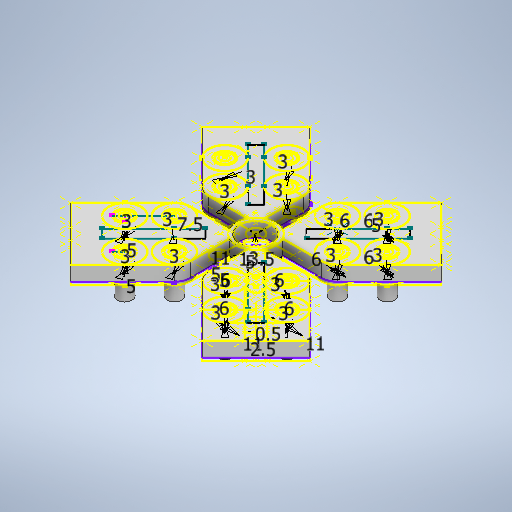
# Autodesk Inventor part: Gripper_Gen3_Base
Saved by Autodesk Inventor 2025.1 (Build 291241000, 241)
## iProperties
Created: 2024-10-29
Part Number: Gripper_Gen3_Base
Material: Generic
Document SubType Name: Modeling
Designer: m_kni
Density: 1 g/cm^3
Appearance: Default
Author: m_kni
Autodesk Inventor part; units mm, degrees
(part 1 of 3)
ref_plane "YZ Plane" through (0, 0, 0) normal (1, 0, 0) x (0, 1, 0)
ref_plane "XZ Plane" through (0, 0, 0) normal (0, 1, 0) x (-1, 0, 0)
ref_plane "XY Plane" through (0, 0, 0) normal (0, 0, 1) x (1, 0, 0)
sketch "Sketch1" plane through (0, 0, 0) normal (0, 1, 0) x (-1, 0, 0)
  arc A0 (-14.3226, 10.9666) -> (-12.7316, 10.3076) centre (-12.7316, 12.5576) ccw
  arc A1 (-14.3226, 10.9666) -> (-12.7316, 10.3076) centre (-12.7316, 12.5576) ccw
  line L0 (-12.7316, 10.3076) -> (-12.7316, 12.5576)
  line L1 (-12.7316, 10.3076) -> (-12.7316, 12.5576)
  line L2 (-12.7316, 12.5576) -> (-10.4816, 12.5576)
  line L3 (-12.7316, 12.5576) -> (-10.4816, 12.5576)
  arc A2 (-14.3226, 17.3306) -> (-17.5046, 14.1486) centre (-15.9136, 15.7396) ccw
  line L4 (-17.5046, 14.1486) -> (-14.3226, 10.9666)
  line L5 (-11.1407, 14.1486) -> (-14.3226, 17.3306)
  arc A3 (-10.4816, 12.5576) -> (-11.1407, 14.1486) centre (-12.7316, 12.5576) ccw
  arc A4 (-14.3226, 17.3306) -> (-17.5046, 14.1486) centre (-15.9136, 15.7396) ccw
  line L6 (-22.9847, 25.9926) -> (-14.3226, 17.3306)
  line L7 (-17.5046, 14.1486) -> (-26.1667, 22.8107)
  arc A5 (-10.4816, 12.5576) -> (-11.1407, 14.1486) centre (-12.7316, 12.5576) ccw
  line L8 (-26.1667, 22.8107) -> (-14.3226, 10.9666)
  line L9 (-26.1667, 22.8107) -> (-14.3226, 10.9666)
  line L10 (-25.9899, 22.9874) -> (-26.1667, 22.8107)
  line L11 (-22.9847, 25.9926) -> (-26.1667, 22.8107)
  line L12 (-26.1667, 22.8107) -> (-22.9847, 25.9926)
  line L13 (-11.1407, 14.1486) -> (-22.9847, 25.9926)
  arc A6 (-10.5886, 13.2429) -> (-11.1407, 14.1486) centre (-12.7316, 12.5576) ccw
  arc A7 (-14.3226, 10.9666) -> (-13.417, 10.4145) centre (-12.7316, 12.5576) ccw
  line L14 (-23.1615, 25.8159) -> (-10.5886, 13.2429)
  line L15 (-22.9847, 25.9926) -> (-11.1407, 14.1486)
  line L16 (-23.1615, 25.8159) -> (-22.9847, 25.9926)
  line L17 (-25.9899, 22.9874) -> (-13.417, 10.4145)
  line L18 (-14.3226, 10.9666) -> (-26.1667, 22.8107)
  line L19 (-26.1667, 22.8107) -> (-25.9899, 22.9874)
  arc A8 (-14.3226, 10.9666) -> (-13.417, 10.4145) centre (-12.7316, 12.5576) ccw
  arc A9 (-10.5886, 13.2429) -> (-11.1407, 14.1486) centre (-12.7316, 12.5576) ccw
  line L20 (-23.1615, 25.8159) -> (-10.5886, 13.2429)
  line L21 (-11.1407, 14.1486) -> (-22.9847, 25.9926)
  line L22 (-22.9847, 25.9926) -> (-23.1615, 25.8159)
  circle A10 centre (-19.2671, 8.4864) radius 2.5
  circle A11 centre (-19.2671, 8.4864) radius 2.5
  circle A12 centre (-17.1458, 27.5783) radius 2.5
  circle A13 centre (-17.1458, 27.5783) radius 2.5
  circle A14 centre (-8.6605, 19.0931) radius 5.5
  circle A15 centre (-27.7524, 16.9717) radius 2.5
  circle A16 centre (-27.7524, 16.9717) radius 2.5
  line L23 (-20.5045, 20.3305) -> (-23.3382, 23.1642)
  arc A17 (-14.3226, 17.3306) -> (-18.0567, 15.0542) centre (-15.9136, 15.7396) ccw
  line L24 (-12.7316, 10.3076) -> (-12.7316, 12.5576)
  line L25 (-12.7316, 12.5576) -> (-10.4816, 12.5576)
  arc A18 (-14.3226, 10.9666) -> (-12.7316, 10.3076) centre (-12.7316, 12.5576) ccw
  arc A19 (-10.4816, 12.5576) -> (-11.1407, 14.1486) centre (-12.7316, 12.5576) ccw
  line L26 (-27.7524, 16.9717) -> (-31.6415, 13.0826)
  line L27 (-31.6415, 13.0826) -> (-23.1562, 4.5974)
  line L28 (-17.1458, 27.5783) -> (-13.2567, 31.4674)
  line L29 (-13.2567, 31.4674) -> (-4.7714, 22.9821)
  circle A20 centre (-0.0316, 12.5576) radius 2.5
  line L30 (-20.5045, 20.3305) -> (-23.3382, 23.1642)
  line L31 (-6.1605, 19.0931) -> (-3.1605, 19.0931)
  line L32 (-3.1605, 19.0931) -> (-3.1605, 12.6302)
  circle A21 centre (-0.0316, -0.1424) radius 6.75
  circle A22 centre (-0.0316, -0.1424) radius 2.5
  line L33 (-3.1605, 12.6302) -> (-3.1605, 5.8386)
  line L34 (-0.0316, -0.1424) -> (-12.7316, -0.1424)
  line L35 (-0.0316, -0.1424) -> (-0.0316, 12.5576)
  line L36 (-0.0316, -0.1424) -> (12.6684, -0.1424)
  line L37 (-19.2671, 2.9864) -> (-6.0127, 2.9864)
  circle A23 centre (-0.0316, -0.1424) radius 2.5
  line L38 (-0.0316, -0.1424) -> (-0.0316, -12.8424)
  line L39 (-20.5045, 24.2196) -> (-13.9798, 17.6948)
  line L40 (-24.3936, 20.3305) -> (-29.7263, 25.6631)
  line L41 (-24.3936, 20.3305) -> (-16.8521, 20.3305) construction
  line L42 (-20.5045, 24.2196) -> (-25.8372, 29.5522)
  line L43 (-29.7263, 25.6631) -> (-33.6153, 29.5522)
  line L44 (-33.6153, 29.5522) -> (-29.7263, 33.4413)
  line L45 (-29.7263, 33.4413) -> (-25.9899, 29.7049)
  line L46 (-21.0349, 31.4674) -> (-24.3936, 28.1087)
  line L47 (-28.2827, 24.2196) -> (-31.6415, 20.8608)
  line L48 (-25.9899, 29.7049) -> (-25.8372, 29.5522)
  line L49 (-23.3382, 23.1642) -> (-31.6708, 31.4968)
  line L50 (-29.1708, 28.9968) -> (-27.2263, 30.9413)
  line L51 (-27.2263, 30.9413) -> (-31.1153, 27.0522)
  line L52 (-33.6153, 29.5522) -> (-40.8632, 22.3044)
  line L53 (-31.6415, 13.0826) -> (-40.8632, 22.3044)
  line L54 (-29.7263, 33.4413) -> (-22.4784, 40.6891)
  line L55 (-13.2567, 31.4674) -> (-22.4784, 40.6891)
  line L56 (-14.3226, 10.9666) -> (-7.0028, 3.6467)
  line L57 (-14.3226, 10.9666) -> (-3.9708, 10.9666) construction
  line L58 (-7.0028, 3.6467) -> (-6.3425, 2.9864)
  line L59 (31.5782, 13.0826) -> (40.7999, 22.3044)
  line L60 (31.5782, 13.0826) -> (23.0929, 4.5974)
  line L61 (33.5521, 29.5522) -> (40.7999, 22.3044)
  line L62 (33.5521, 29.5522) -> (29.663, 33.4413)
  line L63 (29.663, 33.4413) -> (22.4151, 40.6891)
  line L64 (13.1934, 31.4674) -> (22.4151, 40.6891)
  line L65 (13.1934, 31.4674) -> (4.7081, 22.9821)
  line L66 (19.2038, 2.9864) -> (5.9494, 2.9864)
  line L67 (3.0972, 12.6302) -> (3.0972, 5.8386)
  line L68 (3.0972, 19.0931) -> (3.0972, 12.6302)
  line L69 (-17.1458, 27.5783) -> (-22.4491, 22.275)
  line L70 (-23.8633, 20.8608) -> (-27.7524, 16.9717)
  line L71 (-24.3936, 20.3305) -> (-22.4331, 18.3699)
  line L72 (-17.4993, 10.2542) -> (-23.1562, 4.5974)
  arc A24 (-23.1562, 4.5974) -> (-14.3956, 11.0396) centre (-19.2671, 8.4864) ccw
  arc A25 (-15.378, 12.3755) -> (-15.569, 12.5576) centre (-19.2671, 8.4864) ccw
  arc A26 (-15.378, 12.3755) -> (-15.569, 12.5576) centre (-19.2671, 8.4864) ccw
  line L73 (-14.3226, 10.9666) -> (-14.3956, 11.0396)
  line L74 (-15.5548, 12.1988) -> (-15.9136, 12.5576)
  line L75 (-12.3728, 15.3807) -> (-12.5496, 15.204)
  line L76 (-15.378, 12.3755) -> (-15.9083, 11.8452)
  line L77 (-11.1407, 14.1486) -> (-12.3728, 15.3807)
  circle A27 centre (-8.6605, 19.0931) radius 2.5
  circle A28 centre (8.5972, 19.0931) radius 2.5
  circle A29 centre (8.5972, 19.0931) radius 5.5
  arc A30 (14.3323, 11.0396) -> (23.0929, 4.5974) centre (19.2038, 8.4864) ccw
  circle A31 centre (-17.1458, 27.5783) radius 5.5
  circle A32 centre (-27.7524, 16.9717) radius 5.5
  circle A33 centre (27.6891, 16.9717) radius 5.5
  circle A34 centre (17.0825, 27.5783) radius 5.5
  arc A35 (14.3323, 11.0396) -> (23.0929, 4.5974) centre (19.2038, 8.4864) ccw
  circle A36 centre (19.2038, 8.4864) radius 5.5
  circle A37 centre (19.2038, 8.4864) radius 2.5
  circle A38 centre (27.6891, 16.9717) radius 2.5
  circle A39 centre (17.0825, 27.5783) radius 2.5
  line L78 (3.0972, 19.0931) -> (3.0972, 12.6302)
  line L79 (6.0972, 19.0931) -> (3.0972, 19.0931)
  line L80 (-31.6415, 13.0826) -> (-40.8632, 22.3044)
  line L81 (-33.6153, 29.5522) -> (-40.8632, 22.3044)
  circle A40 centre (-17.1458, 27.5783) radius 5.5
  line L82 (-33.6153, 29.5522) -> (-29.7263, 33.4413)
  line L83 (-29.7263, 33.4413) -> (-22.4784, 40.6891)
  line L84 (-13.2567, 31.4674) -> (-22.4784, 40.6891)
  circle A41 centre (-17.1458, 27.5783) radius 2.5
  line L85 (-31.6415, 13.0826) -> (-23.1562, 4.5974)
  line L86 (-13.2567, 31.4674) -> (-4.7714, 22.9821)
  circle A42 centre (-27.7524, 16.9717) radius 5.5
  circle A43 centre (-27.7524, 16.9717) radius 2.5
  circle A44 centre (-8.6605, 19.0931) radius 2.5
  circle A45 centre (-8.6605, 19.0931) radius 5.5
  line L87 (-3.1605, 19.0931) -> (-3.1605, 12.6302)
  circle A46 centre (-19.2671, 8.4864) radius 2.5
  circle A47 centre (-19.2671, 8.4864) radius 5.5
  arc A48 (-23.1562, 4.5974) -> (-14.3956, 11.0396) centre (-19.2671, 8.4864) ccw
  arc A49 (-23.1562, 4.5974) -> (-14.3956, 11.0396) centre (-19.2671, 8.4864) ccw
  line L88 (-19.2671, 2.9864) -> (-6.0127, 2.9864)
  circle A50 centre (-0.0316, 12.5576) radius 2.5
  line L89 (3.0972, 12.6302) -> (3.0972, 5.8386)
  line L90 (-0.0316, -0.1424) -> (-12.7316, -0.1424)
  line L91 (6.9395, 3.6467) -> (6.2792, 2.9864)
  line L92 (-3.1605, 12.6302) -> (-3.1605, 5.8386)
  line L93 (-0.0316, -0.1424) -> (12.6684, -0.1424)
  circle A51 centre (-0.0316, -0.1424) radius 2.5
  circle A52 centre (-0.0316, -0.1424) radius 2.5
  line L94 (31.5782, -13.3674) -> (23.0929, -4.8822)
  circle A53 centre (19.2038, -8.7712) radius 2.5
  circle A54 centre (19.2038, -8.7712) radius 5.5
  arc A55 (23.0929, -4.8822) -> (14.3323, -11.3243) centre (19.2038, -8.7712) ccw
  arc A56 (23.0929, -4.8822) -> (14.3323, -11.3243) centre (19.2038, -8.7712) ccw
  line L95 (-0.0316, -0.1424) -> (-0.0316, -12.8424)
  circle A57 centre (-0.0316, -12.8424) radius 2.5
  line L96 (19.2038, -3.2712) -> (5.9494, -3.2712)
  line L97 (3.0972, -12.915) -> (3.0972, -6.1234)
  line L98 (3.0972, -19.3778) -> (3.0972, -12.915)
  circle A58 centre (8.5972, -19.3778) radius 2.5
  circle A59 centre (8.5972, -19.3778) radius 5.5
  line L99 (6.9395, -3.9315) -> (6.2792, -3.2712)
  line L100 (3.0972, -12.915) -> (3.0972, -6.1234)
  line L101 (3.0972, -19.3778) -> (3.0972, -12.915)
  circle A60 centre (-0.0316, -12.8424) radius 2.5
  line L102 (6.0972, -19.3778) -> (3.0972, -19.3778)
  circle A61 centre (27.6891, -17.2565) radius 2.5
  circle A62 centre (27.6891, -17.2565) radius 5.5
  line L103 (31.5782, -13.3674) -> (40.7999, -22.5892)
  line L104 (33.5521, -29.837) -> (40.7999, -22.5892)
  circle A63 centre (17.0825, -27.8631) radius 2.5
  line L105 (13.1934, -31.7522) -> (4.7081, -23.2669)
  circle A64 centre (17.0825, -27.8631) radius 5.5
  line L106 (33.5521, -29.837) -> (29.663, -33.7261)
  line L107 (13.1934, -31.7522) -> (22.4151, -40.9739)
  line L108 (29.663, -33.7261) -> (22.4151, -40.9739)
  line L109 (-3.1605, -12.915) -> (-3.1605, -6.1234)
  line L110 (-3.1605, -12.915) -> (-3.1605, -6.1234)
  line L111 (-6.1605, -19.3778) -> (-3.1605, -19.3778)
  line L112 (-3.1605, -19.3778) -> (-3.1605, -12.915)
  circle A65 centre (-19.2671, -8.7712) radius 2.5
  line L113 (-31.6415, -13.3674) -> (-23.1562, -4.8822)
  line L114 (-3.1605, -19.3778) -> (-3.1605, -12.915)
  circle A66 centre (-8.6605, -19.3778) radius 2.5
  circle A67 centre (-8.6605, -19.3778) radius 5.5
  line L115 (-13.2567, -31.7522) -> (-4.7714, -23.2669)
  circle A68 centre (-17.1458, -27.8631) radius 2.5
  circle A69 centre (-27.7524, -17.2565) radius 2.5
  circle A70 centre (-17.1458, -27.8631) radius 5.5
  circle A71 centre (-27.7524, -17.2565) radius 5.5
  line L116 (-13.2567, -31.7522) -> (-22.4784, -40.9739)
  line L117 (-31.6415, -13.3674) -> (-40.8632, -22.5892)
  line L118 (-29.7263, -33.7261) -> (-22.4784, -40.9739)
  line L119 (-33.6153, -29.837) -> (-29.7263, -33.7261)
  line L120 (-33.6153, -29.837) -> (-40.8632, -22.5892)
  line L121 (-19.2671, -3.2712) -> (-6.0127, -3.2712)
  arc A72 (-14.3956, -11.3243) -> (-23.1562, -4.8822) centre (-19.2671, -8.7712) ccw
  circle A73 centre (-19.2671, -8.7712) radius 5.5
  circle A74 centre (-0.0316, -0.1424) radius 5.5
  circle A75 centre (-19.2671, 8.4864) radius 3
  circle A76 centre (-8.6605, 19.0931) radius 3
  circle A77 centre (-27.7524, 16.9717) radius 3
  circle A78 centre (-17.1458, 27.5783) radius 3
  point P0 (0, 0)
  point P1 (-17.5046, 17.3306)
  point P2 (-11.1407, 14.1486)
  point P3 (-14.3226, 17.3306)
  point P4 (-17.5046, 14.1486)
  point P5 (-17.5046, 17.3306)
  point P6 (-10.4816, 12.5576)
  point P7 (-12.7316, 12.5576)
  point P8 (-10.4816, 12.5576)
  point P9 (-12.7316, 10.3076)
  point P10 (-15.9136, 15.7396)
  point P11 (17.4413, 14.1486)
  point P12 (25.9266, 22.9874)
  point P13 (-14.3226, -17.6154)
  point P14 (-17.5046, -14.4334)
  point P15 (-11.1407, -14.4334)
  point P16 (-25.9899, -23.2722)
  point P17 (-23.3382, -23.449)
  point P18 (25.9266, -23.2722)
  point P19 (-20.2447, 16.8886)
  point P20 (-12.0192, 15.7343)
  point P21 (4.7081, 22.9821)
  point P22 (3.9075, 10.9666)
  point P23 (3.9075, -11.2514)
  point P24 (4.7081, -23.2669)
  point P25 (25.9266, -23.2722)
  point P26 (17.4413, -14.4334)
  point P27 (-3.9708, -11.2514)
  point P28 (-4.7714, -23.2669)
  point P29 (-17.5046, -14.4334)
  point P30 (-25.9899, -23.2722)
  point P31 (-25.9899, -23.2722)
  point P32 (-3.1605, 19.0931)
  point P33 (-13.532, 16.5399)
  point P34 (-11.2136, 14.2215)
  point P35 (-22.4651, 26.1801)
  point P36 (-18.544, 22.259)
  point P37 (-26.3542, 22.291)
  point P38 (-14.3956, -11.3243)
  point P39 (-14.3956, 11.0396)
  point P40 (-16.714, 13.358)
  point P41 (14.3323, 11.0396)
  point P42 (-14.3956, 11.0396)
  point P43 (-15.378, 12.3755)
  point P44 (-15.569, 12.5576)
  dimension "d0" = 5
  dimension "d1" = 13.5
  dimension "d2" = 5
  dimension "d3" = 0.5
  dimension "d4" = 2.5
  dimension "d5" = 5
  dimension "d6" = 11
  dimension "d7" = 11
  dimension "d8" = 5
  dimension "d9" = 5
  dimension "d10" = 11
  dimension "d40" = 6
  dimension "d41" = 6
  dimension "d42" = 6
  dimension "d43" = 6
  constraints: 244 end point, 121 symmetric about line, 78 centre point, 50 point on circle, 29 coincident, 19 point on line, 9 perpendicular, 6 horizontal, 3 parallel, 3 vertical, 2 equal length, 2 midpoint, 2 tangent, 1 collinear, 1 concentric, 69 other
  measures "d0" diameter of A20
  measures "d1" diameter of A21
  measures "d2" diameter of A22
  measures "d3" distance between parallel lines of L7 L40
  measures "d4" horizontal distance of L50.start L49.end
  measures "d5" diameter of A27
  measures "d6" diameter of A31
  measures "d7" diameter of A32
  measures "d8" diameter of A38
  measures "d9" diameter of A39
  measures "d10" diameter of A74
  measures "d40" diameter of A75
  measures "d41" diameter of A76
  measures "d42" diameter of A77
  measures "d43" diameter of A78
extrude "Extrusion1" add sketch "Sketch1" along normal blind 5 contours L4 A47 L17 A0 | L56 L58 L37 A24 L4 | A0 L0 L2 A3 L5 A14 L32 L33 A21 L37 L58 L56 | L17 A2 L14 A3 L2 L0 A0 | A10 L72 | L72 A10 | A75 | A24 A47 L4 | L4 L76 A47 | A25 A47 L4 A2 L17 | L76 L4 A47 A25 | L17 L11 L49 L23 L69 L14 A2 | A2 L7 A32 L17 | A21 L35 A74 L34 | L4 A47 L27 A32 L7 | L14 A31 L6 A2 | A2 L5 A14 L14 | A32 L7 L10 L17 | A32 L7 L70 | L70 L7 A32 | L34 A74 L38 A21 | L14 A14 L5 A3 | A32 L71 L70 L7 | L6 A31 L39 A14 L5 | L69 L23 L49 L11 L14 | A31 L6 L69 | L14 L11 L6 A31 | L69 L6 A31 | L75 L5 A14 | A14 L5 L75 | L10 L7 A32 L40 L43 L51 L49 L11 | L70 L40 A32 L7 | A32 L40 L70 A77 L26 | L53 L52 L43 L40 L47 A32 | L26 A77 L70 L71 A32 | A21 L36 A74 L35 | A71 | A70 | A21 L109 L112 A67 L115 L116 L118 L119 L120 L117 L113 A73 A72 L121 | A74 L35 A22 L34 | L34 A22 L38 A74 | A27 | A76 | A14 L5 | L6 L69 L39 A31 | L11 L49 L50 L45 L48 L42 A31 L6 | L6 A31 L42 L69 | A32 L47 L40 | A77 L70 A15 L26 | L26 A15 L70 A77 | A33 | A34 | L67 L68 A29 L65 L64 L63 L62 L61 L59 L60 A36 A30 L66 A21 | A74 L36 A22 L35 | A72 A73 | L34 L38 A22 | A22 L35 L34 | A74 L36 A21 L38 | L38 A22 L36 A74 | L39 A31 L29 A14 | L39 L69 A78 L28 A31 | L42 A31 L28 A78 L69 | L42 L46 A31 | L51 L43 L44 L49 | L49 L44 L45 L50 | L26 L70 A15 | A15 L70 L26 | A22 L36 L35 | L38 L36 A22 | A78 L28 A12 L69 | L69 A12 L28 A78 | L42 L48 L45 L54 L55 A31 L46 | A29 | A28 | A64 | A62 | A21 L96 A54 L94 L103 L104 L106 L108 L107 L105 A59 L98 L97 | A66 | A67 | L69 L28 A12 | A12 L28 L69 | A30 A36 | A59 | A58 | A54 | A37 | A38 | A39 | A53 | A61 | A63 | A65 | A68 | A69
extrude "Extrusion2" add sketch "Sketch1" against normal blind 1 contours A10 L72 | L72 A10 | A75 | A24 A47 L4 | L4 L76 A47 | L76 L4 A47 A25 | L75 L5 A14 | A14 L5 L75 | A32 L40 L70 A77 L26 | L26 A77 L70 L71 A32 | A71 | A70 | A27 | A76 | A14 L5 | A77 L70 A15 L26 | L26 A15 L70 A77 | A33 | A34 | A72 A73 | L39 L69 A78 L28 A31 | L42 A31 L28 A78 L69 | L26 L70 A15 | A15 L70 L26 | A78 L28 A12 L69 | L69 A12 L28 A78 | A29 | A28 | A64 | A62 | A66 | A67 | L69 L28 A12 | A12 L28 L69 | A30 A36 | A59 | A58 | A54 | A37 | A38 | A39 | A53 | A61 | A63 | A65 | A68 | A69
sketch "Sketch3" plane through (17.1458, -1, -27.8631) normal (0, -1, 0) x (1, 0, 0)
  circle A0 centre (0, 0) radius 2.5
  arc A1 (-11.1331, 24.5919) -> (-11.1331, 30.8496) centre (-17.1141, 27.7207) ccw projected
  line L0 (2.1213, 30.8496) -> (-11.1331, 30.8496) projected
  line L1 (-11.1331, 24.5919) -> (2.1213, 24.5919) projected
  arc A2 (2.1213, 30.8496) -> (6.0104, 32.4605) centre (2.1213, 36.3496) ccw projected
  line L2 (6.0104, 22.981) -> (23.7174, 5.274) projected
  arc A3 (6.0104, 22.981) -> (2.1213, 24.5919) centre (2.1213, 19.0919) ccw projected
  arc A4 (-20.243, 21.7397) -> (-13.9853, 21.7397) centre (-17.1141, 27.7207) ccw projected
  line L3 (-13.9853, 8.4853) -> (-13.9853, 21.7397) projected
  arc A5 (-13.9853, 8.4853) -> (-12.3744, 4.5962) centre (-8.4853, 8.4853) ccw projected
  line L4 (5.3326, -13.1108) -> (-12.3744, 4.5962) projected
  line L5 (23.7174, 5.274) -> (5.3326, -13.1108) projected
  line L6 (-20.243, 21.7397) -> (-20.243, 8.4853) projected
  line L7 (-21.8539, 4.5962) -> (-39.5609, -13.1108) projected
  line L8 (-39.5609, -13.1108) -> (-57.9457, 5.274) projected
  arc A6 (-21.8539, 4.5962) -> (-20.243, 8.4853) centre (-25.743, 8.4853) ccw projected
  line L9 (-12.3744, 50.8453) -> (5.3326, 68.5523) projected
  line L10 (5.3326, 68.5523) -> (23.7174, 50.1675) projected
  line L11 (23.7174, 50.1675) -> (6.0104, 32.4605) projected
  arc A7 (-13.9853, 33.7018) -> (-20.243, 33.7018) centre (-17.1141, 27.7207) ccw projected
  arc A8 (-13.9853, 33.7018) -> (-20.243, 33.7018) centre (-17.1141, 27.7207) ccw projected
  arc A9 (-13.9853, 33.7018) -> (-20.243, 33.7018) centre (-17.1141, 27.7207) ccw projected
  arc A10 (-13.9853, 33.7018) -> (-20.243, 33.7018) centre (-17.1141, 27.7207) ccw projected
  line L12 (-13.9853, 33.7018) -> (-13.9853, 46.9562) projected
  line L13 (-12.3744, 50.8453) -> (5.3326, 68.5523) projected
  line L14 (5.3326, 68.5523) -> (23.7174, 50.1675) projected
  line L15 (23.7174, 50.1675) -> (6.0104, 32.4605) projected
  arc A11 (2.1213, 30.8496) -> (6.0104, 32.4605) centre (2.1213, 36.3496) ccw projected
  line L16 (2.1213, 30.8496) -> (-11.1331, 30.8496) projected
  arc A12 (-11.1331, 24.5919) -> (-11.1331, 30.8496) centre (-17.1141, 27.7207) ccw projected
  line L17 (-11.1331, 24.5919) -> (2.1213, 24.5919) projected
  arc A13 (6.0104, 22.981) -> (2.1213, 24.5919) centre (2.1213, 19.0919) ccw projected
  line L18 (6.0104, 22.981) -> (23.7174, 5.274) projected
  line L19 (23.7174, 5.274) -> (5.3326, -13.1108) projected
  line L20 (5.3326, -13.1108) -> (-12.3744, 4.5962) projected
  arc A14 (-13.9853, 8.4853) -> (-12.3744, 4.5962) centre (-8.4853, 8.4853) ccw projected
  line L21 (-13.9853, 8.4853) -> (-13.9853, 21.7397) projected
  arc A15 (-20.243, 21.7397) -> (-13.9853, 21.7397) centre (-17.1141, 27.7207) ccw projected
  line L22 (-20.243, 21.7397) -> (-20.243, 8.4853) projected
  arc A16 (-21.8539, 4.5962) -> (-20.243, 8.4853) centre (-25.743, 8.4853) ccw projected
  line L23 (-21.8539, 4.5962) -> (-39.5609, -13.1108) projected
  line L24 (-39.5609, -13.1108) -> (-57.9457, 5.274) projected
  line L25 (-57.9457, 5.274) -> (-40.2387, 22.981) projected
  arc A17 (-36.3496, 24.5919) -> (-40.2387, 22.981) centre (-36.3496, 19.0919) ccw projected
  line L26 (-36.3496, 24.5919) -> (-23.0952, 24.5919) projected
  arc A18 (-23.0952, 30.8496) -> (-23.0952, 24.5919) centre (-17.1141, 27.7207) ccw projected
  line L27 (-23.0952, 30.8496) -> (-36.3496, 30.8496) projected
  arc A19 (-40.2387, 32.4605) -> (-36.3496, 30.8496) centre (-36.3496, 36.3496) ccw projected
  line L28 (-40.2387, 32.4605) -> (-57.9457, 50.1675) projected
  line L29 (-57.9457, 50.1675) -> (-39.5609, 68.5523) projected
  line L30 (-39.5609, 68.5523) -> (-21.8539, 50.8453) projected
  arc A20 (-20.243, 46.9562) -> (-21.8539, 50.8453) centre (-25.743, 46.9562) ccw projected
  line L31 (-20.243, 46.9562) -> (-20.243, 33.7018) projected
  arc A21 (-13.9853, 33.7018) -> (-20.243, 33.7018) centre (-17.1141, 27.7207) ccw projected
  line L32 (-13.9853, 33.7018) -> (-13.9853, 46.9562) projected
  arc A22 (-12.3744, 50.8453) -> (-13.9853, 46.9562) centre (-8.4853, 46.9562) ccw projected
  arc A23 (2.1213, 24.5919) -> (6.0104, 22.981) centre (2.1213, 19.0919) ccw projected
  line L33 (-11.1331, 24.5919) -> (2.1213, 24.5919) projected
  arc A24 (-11.1331, 24.5919) -> (-11.1331, 30.8496) centre (-17.1141, 27.7207) ccw projected
  line L34 (2.1213, 30.8496) -> (-11.1331, 30.8496) projected
  arc A25 (6.0104, 32.4605) -> (2.1213, 30.8496) centre (2.1213, 36.3496) ccw projected
  line L35 (14.4957, 40.9458) -> (6.0104, 32.4605) projected
  arc A26 (5.2873, 46.2331) -> (14.4957, 40.9458) centre (10.6066, 44.8349) ccw projected
  line L36 (5.2873, 46.2331) -> (9.2084, 50.1542) projected
  arc A27 (14.4957, 40.9458) -> (9.2084, 50.1542) centre (10.6066, 44.8349) ccw projected
  line L37 (23.7174, 50.1675) -> (14.4957, 40.9458) projected
  line L38 (5.3326, 68.5523) -> (23.7174, 50.1675) projected
  line L39 (-3.8891, 59.3305) -> (5.3326, 68.5523) projected
  arc A28 (5.3193, 54.0432) -> (-3.8891, 59.3305) centre (0, 55.4415) ccw projected
  line L40 (5.3193, 54.0432) -> (1.3982, 50.1222) projected
  arc A29 (-3.8891, 59.3305) -> (1.3982, 50.1222) centre (0, 55.4415) ccw projected
  line L41 (-12.3744, 50.8453) -> (-3.8891, 59.3305) projected
  arc A30 (-13.9853, 46.9562) -> (-12.3744, 50.8453) centre (-8.4853, 46.9562) ccw projected
  line L42 (-13.9853, 33.7018) -> (-13.9853, 46.9562) projected
  arc A31 (-13.9853, 33.7018) -> (-20.243, 33.7018) centre (-17.1141, 27.7207) ccw projected
  line L43 (-20.243, 46.9562) -> (-20.243, 33.7018) projected
  arc A32 (-21.8539, 50.8453) -> (-20.243, 46.9562) centre (-25.743, 46.9562) ccw projected
  line L44 (-30.3392, 59.3305) -> (-21.8539, 50.8453) projected
  circle A33 centre (-34.2283, 55.4415) radius 5.5 projected
  line L45 (-39.5609, 68.5523) -> (-30.3392, 59.3305) projected
  line L46 (-57.9457, 50.1675) -> (-39.5609, 68.5523) projected
  line L47 (-48.7239, 40.9458) -> (-57.9457, 50.1675) projected
  circle A34 centre (-44.8349, 44.8349) radius 5.5 projected
  line L48 (-40.2387, 32.4605) -> (-48.7239, 40.9458) projected
  arc A35 (-36.3496, 30.8496) -> (-40.2387, 32.4605) centre (-36.3496, 36.3496) ccw projected
  line L49 (-23.0952, 30.8496) -> (-36.3496, 30.8496) projected
  arc A36 (-23.0952, 30.8496) -> (-23.0952, 24.5919) centre (-17.1141, 27.7207) ccw projected
  line L50 (-36.3496, 24.5919) -> (-23.0952, 24.5919) projected
  arc A37 (-40.2387, 22.981) -> (-36.3496, 24.5919) centre (-36.3496, 19.0919) ccw projected
  line L51 (-48.7239, 14.4957) -> (-40.2387, 22.981) projected
  circle A38 centre (-44.8349, 10.6066) radius 5.5 projected
  line L52 (-57.9457, 5.274) -> (-48.7239, 14.4957) projected
  line L53 (-39.5609, -13.1108) -> (-57.9457, 5.274) projected
  line L54 (-30.3392, -3.8891) -> (-39.5609, -13.1108) projected
  circle A39 centre (-34.2283, 0) radius 5.5 projected
  line L55 (-21.8539, 4.5962) -> (-30.3392, -3.8891) projected
  arc A40 (-20.243, 8.4853) -> (-21.8539, 4.5962) centre (-25.743, 8.4853) ccw projected
  line L56 (-20.243, 21.7397) -> (-20.243, 8.4853) projected
  arc A41 (-20.243, 21.7397) -> (-13.9853, 21.7397) centre (-17.1141, 27.7207) ccw projected
  line L57 (-13.9853, 8.4853) -> (-13.9853, 21.7397) projected
  arc A42 (-12.3744, 4.5962) -> (-13.9853, 8.4853) centre (-8.4853, 8.4853) ccw projected
  line L58 (-3.8891, -3.8891) -> (-12.3744, 4.5962) projected
  circle A43 centre (0, 0) radius 5.5 projected
  line L59 (5.3326, -13.1108) -> (-3.8891, -3.8891) projected
  line L60 (23.7174, 5.274) -> (5.3326, -13.1108) projected
  line L61 (14.4957, 14.4957) -> (23.7174, 5.274) projected
  circle A44 centre (10.6066, 10.6066) radius 5.5 projected
  line L62 (6.0104, 22.981) -> (14.4957, 14.4957) projected
  line L63 (-20.243, 46.9562) -> (-20.243, 33.7018) projected
  line L64 (-20.243, 46.9562) -> (-20.243, 33.7018) projected
  arc A45 (-20.243, 46.9562) -> (-21.8539, 50.8453) centre (-25.743, 46.9562) ccw projected
  arc A46 (-40.2387, 32.4605) -> (-36.3496, 30.8496) centre (-36.3496, 36.3496) ccw projected
  arc A47 (-36.3496, 30.8496) -> (-40.2387, 32.4605) centre (-36.3496, 36.3496) ccw projected
  line L65 (-30.3392, 59.3305) -> (-21.8539, 50.8453) projected
  line L66 (-40.2387, 32.4605) -> (-48.7239, 40.9458) projected
  line L67 (-39.5609, 68.5523) -> (-21.8539, 50.8453) projected
  line L68 (-39.5609, 68.5523) -> (-30.3392, 59.3305) projected
  line L69 (-40.2387, 32.4605) -> (-57.9457, 50.1675) projected
  line L70 (-48.7239, 40.9458) -> (-57.9457, 50.1675) projected
  arc A48 (-21.8539, 50.8453) -> (-20.243, 46.9562) centre (-25.743, 46.9562) ccw projected
  line L71 (-23.0952, 30.8496) -> (-36.3496, 30.8496) projected
  arc A49 (-23.0952, 30.8496) -> (-23.0952, 24.5919) centre (-17.1141, 27.7207) ccw projected
  line L72 (-36.3496, 24.5919) -> (-23.0952, 24.5919) projected
  arc A50 (-36.3496, 24.5919) -> (-40.2387, 22.981) centre (-36.3496, 19.0919) ccw projected
  line L73 (-57.9457, 5.274) -> (-40.2387, 22.981) projected
  line L74 (-23.0952, 30.8496) -> (-36.3496, 30.8496) projected
  line L75 (-23.0952, 30.8496) -> (-36.3496, 30.8496) projected
  arc A51 (-12.3744, 50.8453) -> (-13.9853, 46.9562) centre (-8.4853, 46.9562) ccw projected
  line L76 (-57.9457, 50.1675) -> (-39.5609, 68.5523) projected
  line L77 (-23.0952, 30.8496) -> (-36.3496, 30.8496) projected
  line L78 (-48.7239, 14.4957) -> (-40.2387, 22.981) projected
  line L79 (-57.9457, 5.274) -> (-48.7239, 14.4957) projected
  arc A52 (-20.243, 8.4853) -> (-21.8539, 4.5962) centre (-25.743, 8.4853) ccw projected
  line L80 (-39.5609, -13.1108) -> (-57.9457, 5.274) projected
  line L81 (-30.3392, -3.8891) -> (-39.5609, -13.1108) projected
  line L82 (-21.8539, 4.5962) -> (-30.3392, -3.8891) projected
  line L83 (-13.9853, 8.4853) -> (-13.9853, 21.7397) projected
  arc A53 (-20.243, 21.7397) -> (-13.9853, 21.7397) centre (-17.1141, 27.7207) ccw projected
  line L84 (-13.9853, 8.4853) -> (-13.9853, 21.7397) projected
  line L85 (-13.9853, 8.4853) -> (-13.9853, 21.7397) projected
  arc A54 (-20.243, 21.7397) -> (-13.9853, 21.7397) centre (-17.1141, 27.7207) ccw projected
  arc A55 (-20.243, 21.7397) -> (-13.9853, 21.7397) centre (-17.1141, 27.7207) ccw projected
  line L86 (-20.243, 21.7397) -> (-20.243, 8.4853) projected
  line L87 (-20.243, 21.7397) -> (-20.243, 8.4853) projected
  line L88 (-20.243, 21.7397) -> (-20.243, 8.4853) projected
  arc A56 (-23.0952, 30.8496) -> (-23.0952, 24.5919) centre (-17.1141, 27.7207) ccw projected
  arc A57 (-12.3744, 4.5962) -> (-13.9853, 8.4853) centre (-8.4853, 8.4853) ccw projected
  line L89 (-3.8891, -3.8891) -> (-12.3744, 4.5962) projected
  line L90 (5.3326, -13.1108) -> (-3.8891, -3.8891) projected
  line L91 (6.0104, 22.981) -> (14.4957, 14.4957) projected
  line L92 (23.7174, 5.274) -> (5.3326, -13.1108) projected
  line L93 (14.4957, 14.4957) -> (23.7174, 5.274) projected
  arc A58 (-23.0952, 30.8496) -> (-23.0952, 24.5919) centre (-17.1141, 27.7207) ccw projected
  arc A59 (-23.0952, 30.8496) -> (-23.0952, 24.5919) centre (-17.1141, 27.7207) ccw projected
  line L94 (-57.9457, 50.1675) -> (-39.5609, 68.5523) projected
  line L95 (-36.3496, 24.5919) -> (-23.0952, 24.5919) projected
  arc A60 (-40.2387, 22.981) -> (-36.3496, 24.5919) centre (-36.3496, 19.0919) ccw projected
  circle A61 centre (-36.3496, 19.0919) radius 5.5 projected
  circle A62 centre (-36.3496, 19.0919) radius 5.5 projected
  circle A63 centre (-36.3496, 19.0919) radius 5.5 projected
  arc A64 (-36.3496, 24.5919) -> (-40.2387, 22.981) centre (-36.3496, 19.0919) ccw projected
  arc A65 (-40.2387, 22.981) -> (-36.3496, 24.5919) centre (-36.3496, 19.0919) ccw projected
  line L96 (-36.3496, 24.5919) -> (-23.0952, 24.5919) projected
  line L97 (-36.3496, 24.5919) -> (-23.0952, 24.5919) projected
  line L98 (-13.9853, 33.7018) -> (-13.9853, 46.9562) projected
  arc A66 (-13.9853, 46.9562) -> (-12.3744, 50.8453) centre (-8.4853, 46.9562) ccw projected
  line L99 (-12.3744, 50.8453) -> (-3.8891, 59.3305) projected
  line L100 (-3.8891, 59.3305) -> (5.3326, 68.5523) projected
  line L101 (5.3326, 68.5523) -> (23.7174, 50.1675) projected
  line L102 (2.1213, 30.8496) -> (-11.1331, 30.8496) projected
  line L103 (2.1213, 30.8496) -> (-11.1331, 30.8496) projected
  line L104 (2.1213, 30.8496) -> (-11.1331, 30.8496) projected
  arc A67 (6.0104, 32.4605) -> (2.1213, 30.8496) centre (2.1213, 36.3496) ccw projected
  circle A68 centre (2.1213, 36.3496) radius 5.5 projected
  arc A69 (2.1213, 30.8496) -> (6.0104, 32.4605) centre (2.1213, 36.3496) ccw projected
  arc A70 (6.0104, 32.4605) -> (2.1213, 30.8496) centre (2.1213, 36.3496) ccw projected
  line L105 (-13.9853, 33.7018) -> (-13.9853, 46.9562) projected
  line L106 (-13.9853, 33.7018) -> (-13.9853, 46.9562) projected
  line L107 (14.4957, 40.9458) -> (6.0104, 32.4605) projected
  circle A71 centre (-8.4853, 46.9562) radius 5.5 projected
  circle A72 centre (-8.4853, 46.9562) radius 5.5 projected
  arc A73 (-12.3744, 50.8453) -> (-13.9853, 46.9562) centre (-8.4853, 46.9562) ccw projected
  arc A74 (-13.9853, 46.9562) -> (-12.3744, 50.8453) centre (-8.4853, 46.9562) ccw projected
  line L108 (23.7174, 50.1675) -> (14.4957, 40.9458) projected
  line L109 (14.4957, 40.9458) -> (6.0104, 32.4605) projected
  line L110 (23.7174, 50.1675) -> (6.0104, 32.4605) projected
  line L111 (23.7174, 50.1675) -> (14.4957, 40.9458) projected
  line L112 (5.3326, 68.5523) -> (23.7174, 50.1675) projected
  line L113 (5.3326, 68.5523) -> (23.7174, 50.1675) projected
  line L114 (-12.3744, 50.8453) -> (-3.8891, 59.3305) projected
  line L115 (-3.8891, 59.3305) -> (5.3326, 68.5523) projected
  line L116 (-12.3744, 50.8453) -> (5.3326, 68.5523) projected
  circle A75 centre (-8.4853, 46.9562) radius 5.5 projected
  arc A76 (-11.1331, 24.5919) -> (-11.1331, 30.8496) centre (-17.1141, 27.7207) ccw projected
  arc A77 (-11.1331, 24.5919) -> (-11.1331, 30.8496) centre (-17.1141, 27.7207) ccw projected
  line L117 (-11.1331, 24.5919) -> (2.1213, 24.5919) projected
  line L118 (-11.1331, 24.5919) -> (2.1213, 24.5919) projected
  line L119 (-11.1331, 24.5919) -> (2.1213, 24.5919) projected
  arc A78 (2.1213, 24.5919) -> (6.0104, 22.981) centre (2.1213, 19.0919) ccw projected
  circle A79 centre (2.1213, 19.0919) radius 5.5 projected
  circle A80 centre (2.1213, 19.0919) radius 5.5 projected
  circle A81 centre (2.1213, 19.0919) radius 5.5 projected
  arc A82 (6.0104, 22.981) -> (2.1213, 24.5919) centre (2.1213, 19.0919) ccw projected
  arc A83 (2.1213, 24.5919) -> (6.0104, 22.981) centre (2.1213, 19.0919) ccw projected
  arc A84 (-11.1331, 24.5919) -> (-11.1331, 30.8496) centre (-17.1141, 27.7207) ccw projected
  line L120 (23.7174, 5.274) -> (5.3326, -13.1108) projected
  line L121 (23.7174, 5.274) -> (5.3326, -13.1108) projected
  line L122 (6.0104, 22.981) -> (14.4957, 14.4957) projected
  line L123 (14.4957, 14.4957) -> (23.7174, 5.274) projected
  line L124 (6.0104, 22.981) -> (23.7174, 5.274) projected
  circle A85 centre (-25.743, 8.4853) radius 5.5 projected
  circle A86 centre (-25.743, 8.4853) radius 5.5 projected
  arc A87 (-21.8539, 4.5962) -> (-20.243, 8.4853) centre (-25.743, 8.4853) ccw projected
  arc A88 (-20.243, 8.4853) -> (-21.8539, 4.5962) centre (-25.743, 8.4853) ccw projected
  line L125 (-21.8539, 4.5962) -> (-30.3392, -3.8891) projected
  line L126 (-30.3392, -3.8891) -> (-39.5609, -13.1108) projected
  line L127 (-21.8539, 4.5962) -> (-39.5609, -13.1108) projected
  line L128 (-39.5609, -13.1108) -> (-57.9457, 5.274) projected
  line L129 (-39.5609, -13.1108) -> (-57.9457, 5.274) projected
  circle A89 centre (-25.743, 8.4853) radius 5.5 projected
  circle A90 centre (-34.2283, 55.4415) radius 5.5 projected
  circle A91 centre (-34.2283, 55.4415) radius 5.5 projected
  circle A92 centre (-36.3496, 36.3496) radius 5.5 projected
  circle A93 centre (-25.743, 46.9562) radius 5.5 projected
  circle A94 centre (-44.8349, 44.8349) radius 5.5 projected
  circle A95 centre (-44.8349, 44.8349) radius 5.5 projected
  line L130 (-20.243, 46.9562) -> (-20.243, 33.7018) projected
  line L131 (-20.243, 46.9562) -> (-20.243, 33.7018) projected
  circle A96 centre (-36.3496, 36.3496) radius 5.5 projected
  arc A97 (-40.2387, 32.4605) -> (-36.3496, 30.8496) centre (-36.3496, 36.3496) ccw projected
  arc A98 (-36.3496, 30.8496) -> (-40.2387, 32.4605) centre (-36.3496, 36.3496) ccw projected
  circle A99 centre (-36.3496, 36.3496) radius 5.5 projected
  circle A100 centre (-25.743, 46.9562) radius 5.5 projected
  circle A101 centre (-34.2283, 55.4415) radius 5.5 projected
  circle A102 centre (-34.2283, 55.4415) radius 5.5 projected
  circle A103 centre (-34.2283, 55.4415) radius 5.5 projected
  circle A104 centre (-44.8349, 44.8349) radius 5.5 projected
  circle A105 centre (-44.8349, 44.8349) radius 5.5 projected
  circle A106 centre (-44.8349, 44.8349) radius 5.5 projected
  line L132 (-40.2387, 32.4605) -> (-48.7239, 40.9458) projected
  line L133 (-48.7239, 40.9458) -> (-57.9457, 50.1675) projected
  line L134 (-40.2387, 32.4605) -> (-57.9457, 50.1675) projected
  line L135 (-57.9457, 50.1675) -> (-39.5609, 68.5523) projected
  line L136 (-57.9457, 50.1675) -> (-39.5609, 68.5523) projected
  circle A107 centre (-25.743, 46.9562) radius 5.5 projected
  arc A108 (-20.243, 46.9562) -> (-21.8539, 50.8453) centre (-25.743, 46.9562) ccw projected
  arc A109 (-21.8539, 50.8453) -> (-20.243, 46.9562) centre (-25.743, 46.9562) ccw projected
  circle A110 centre (0, 0) radius 5.5 projected
  circle A111 centre (0, 0) radius 5.5 projected
  circle A112 centre (10.6066, 10.6066) radius 5.5 projected
  circle A113 centre (10.6066, 10.6066) radius 5.5 projected
  circle A114 centre (0, 0) radius 5.5 projected
  circle A115 centre (0, 0) radius 5.5 projected
  circle A116 centre (0, 0) radius 5.5 projected
  circle A117 centre (10.6066, 10.6066) radius 5.5 projected
  circle A118 centre (10.6066, 10.6066) radius 5.5 projected
  circle A119 centre (10.6066, 10.6066) radius 5.5 projected
  circle A120 centre (-44.8349, 10.6066) radius 5.5 projected
  circle A121 centre (-44.8349, 10.6066) radius 5.5 projected
  circle A122 centre (-34.2283, 0) radius 5.5 projected
  circle A123 centre (-34.2283, 0) radius 5.5 projected
  circle A124 centre (-34.2283, 0) radius 5.5 projected
  circle A125 centre (-34.2283, 0) radius 5.5 projected
  circle A126 centre (-34.2283, 0) radius 5.5 projected
  circle A127 centre (-44.8349, 10.6066) radius 5.5 projected
  circle A128 centre (-44.8349, 10.6066) radius 5.5 projected
  line L137 (-57.9457, 5.274) -> (-48.7239, 14.4957) projected
  line L138 (-48.7239, 14.4957) -> (-40.2387, 22.981) projected
  line L139 (-57.9457, 5.274) -> (-40.2387, 22.981) projected
  circle A129 centre (-44.8349, 10.6066) radius 5.5 projected
  line L140 (-39.5609, 68.5523) -> (-30.3392, 59.3305) projected
  line L141 (-30.3392, 59.3305) -> (-21.8539, 50.8453) projected
  line L142 (-39.5609, 68.5523) -> (-21.8539, 50.8453) projected
  arc A130 (5.2873, 46.2331) -> (14.4957, 40.9458) centre (10.6066, 44.8349) ccw projected
  arc A131 (5.2873, 46.2331) -> (9.2084, 50.1542) centre (10.6066, 44.8349) ccw projected
  arc A132 (14.4957, 40.9458) -> (9.2084, 50.1542) centre (10.6066, 44.8349) ccw projected
  line L143 (9.2084, 50.1542) -> (5.2873, 46.2331) projected
  line L144 (5.2873, 46.2331) -> (9.2084, 50.1542) projected
  line L145 (1.3982, 50.1222) -> (5.3193, 54.0432) projected
  line L146 (5.3193, 54.0432) -> (1.3982, 50.1222) projected
  arc A133 (5.3193, 54.0432) -> (-3.8891, 59.3305) centre (0, 55.4415) ccw projected
  arc A134 (5.3193, 54.0432) -> (1.3982, 50.1222) centre (0, 55.4415) ccw projected
  arc A135 (-3.8891, 59.3305) -> (1.3982, 50.1222) centre (0, 55.4415) ccw projected
  circle A136 centre (2.1213, 36.3496) radius 5.5 projected
  line L147 (5.2873, 46.2331) -> (9.2084, 50.1542) projected
  line L148 (9.2084, 50.1542) -> (5.2873, 46.2331) projected
  line L149 (5.3193, 54.0432) -> (1.3982, 50.1222) projected
  line L150 (1.3982, 50.1222) -> (5.3193, 54.0432) projected
  line L151 (1.3982, 50.1222) -> (5.3193, 54.0432) projected
  arc A137 (5.3193, 54.0432) -> (1.3982, 50.1222) centre (0, 55.4415) ccw projected
  arc A138 (-3.8891, 59.3305) -> (1.3982, 50.1222) centre (0, 55.4415) ccw projected
  arc A139 (5.3193, 54.0432) -> (1.3982, 50.1222) centre (0, 55.4415) ccw projected
  arc A140 (5.3193, 54.0432) -> (-3.8891, 59.3305) centre (0, 55.4415) ccw projected
  arc A141 (14.4957, 40.9458) -> (9.2084, 50.1542) centre (10.6066, 44.8349) ccw projected
  arc A142 (5.2873, 46.2331) -> (9.2084, 50.1542) centre (10.6066, 44.8349) ccw projected
  arc A143 (5.2873, 46.2331) -> (14.4957, 40.9458) centre (10.6066, 44.8349) ccw projected
  arc A144 (5.2873, 46.2331) -> (9.2084, 50.1542) centre (10.6066, 44.8349) ccw projected
  line L152 (9.2084, 50.1542) -> (5.2873, 46.2331) projected
  circle A145 centre (2.1213, 36.3496) radius 5.5 projected
  circle A146 centre (-8.4853, 8.4853) radius 5.5 projected
  circle A147 centre (-8.4853, 8.4853) radius 5.5 projected
  arc A148 (-13.9853, 8.4853) -> (-12.3744, 4.5962) centre (-8.4853, 8.4853) ccw projected
  arc A149 (-12.3744, 4.5962) -> (-13.9853, 8.4853) centre (-8.4853, 8.4853) ccw projected
  line L153 (5.3326, -13.1108) -> (-3.8891, -3.8891) projected
  line L154 (-3.8891, -3.8891) -> (-12.3744, 4.5962) projected
  line L155 (5.3326, -13.1108) -> (-12.3744, 4.5962) projected
  circle A150 centre (-8.4853, 8.4853) radius 5.5 projected
  circle A151 centre (-44.8349, 44.8349) radius 2.5 projected
  circle A152 centre (-44.8349, 44.8349) radius 5.5 projected
  line L156 (-30.3392, 59.3305) -> (-21.8539, 50.8453) projected
  circle A153 centre (-34.2283, 55.4415) radius 2.5 projected
  circle A154 centre (-34.2283, 55.4415) radius 5.5 projected
  line L157 (-30.3392, 59.3305) -> (-39.5609, 68.5523) projected
  line L158 (-46.8087, 61.3044) -> (-39.5609, 68.5523) projected
  line L159 (-50.6978, 57.4153) -> (-46.8087, 61.3044) projected
  line L160 (-50.6978, 57.4153) -> (-57.9457, 50.1675) projected
  line L161 (-48.7239, 40.9458) -> (-57.9457, 50.1675) projected
  arc A155 (0.3588, 42.0117) -> (-2.8231, 45.1937) centre (-1.2321, 43.6027) ccw projected
  line L162 (0.3588, 42.0117) -> (-2.8231, 38.8297) projected
  line L163 (3.3588, 48.1936) -> (6.1925, 51.0273) projected
  line L164 (3.3588, 48.1936) -> (6.1925, 51.0273) projected
  line L165 (7.2478, 48.1936) -> (-0.2937, 48.1936) construction
  line L166 (0.3588, 42.0117) -> (9.0209, 50.6738) projected
  line L167 (5.8389, 53.8558) -> (-2.8231, 45.1937) projected
  line L168 (3.3588, 52.0827) -> (-3.166, 45.558) projected
  line L169 (9.0209, 50.6738) -> (-2.8231, 38.8297) projected
  line L170 (9.0209, 50.6738) -> (-2.8231, 38.8297) projected
  line L171 (-2.8231, 38.8297) -> (9.0209, 50.6738) projected
  line L172 (8.8441, 50.8506) -> (-3.7288, 38.2776) projected
  line L173 (-6.0051, 42.0117) -> (5.8389, 53.8558) projected
  line L174 (-6.0051, 42.0117) -> (5.8389, 53.8558) projected
  line L175 (5.8389, 53.8558) -> (-6.0051, 42.0117) projected
  line L176 (6.0157, 53.679) -> (-6.5572, 41.1061) projected
  line L177 (6.0157, 53.679) -> (-6.5572, 41.1061) projected
  arc A156 (0.3588, 42.0117) -> (-2.8231, 45.1937) centre (-1.2321, 43.6027) ccw projected
  line L178 (-6.0051, 42.0117) -> (-2.8231, 45.1937) projected
  line L179 (-4.4141, 38.1707) -> (-4.4141, 40.4207) projected
  line L180 (-4.4141, 38.1707) -> (-4.4141, 40.4207) projected
  line L181 (-4.4141, 40.4207) -> (-6.6641, 40.4207) projected
  line L182 (-4.4141, 40.4207) -> (-6.6641, 40.4207) projected
  arc A157 (-6.0051, 42.0117) -> (-6.6641, 40.4207) centre (-4.4141, 40.4207) ccw projected
  arc A158 (-6.0051, 42.0117) -> (-6.6641, 40.4207) centre (-4.4141, 40.4207) ccw projected
  circle A159 centre (-8.4853, 46.9562) radius 2.5 projected
  line L183 (-2.8231, 38.8297) -> (-13.175, 38.8297) construction
  line L184 (-2.8231, 38.8297) -> (-10.143, 31.5099) projected
  line L185 (-13.9853, 40.4933) -> (-13.9853, 33.7018) projected
  line L186 (-13.9853, 46.9562) -> (-13.9853, 40.4933) projected
  line L187 (6.0157, 53.679) -> (5.8389, 53.8558) projected
  line L188 (8.8441, 50.8506) -> (9.0209, 50.6738) projected
  line L189 (9.0209, 50.6738) -> (8.8441, 50.8506) projected
  line L190 (5.8389, 53.8558) -> (9.0209, 50.6738) projected
  line L191 (9.0209, 50.6738) -> (5.8389, 53.8558) projected
  line L192 (-3.8891, 59.3305) -> (5.3326, 68.5523) projected
  line L193 (-3.8891, 59.3305) -> (5.3326, 68.5523) projected
  line L194 (12.5805, 61.3044) -> (5.3326, 68.5523) projected
  line L195 (12.5805, 61.3044) -> (5.3326, 68.5523) projected
  arc A160 (-4.4141, 38.1707) -> (-2.8231, 38.8297) centre (-4.4141, 40.4207) ccw projected
  arc A161 (-4.4141, 38.1707) -> (-2.8231, 38.8297) centre (-4.4141, 40.4207) ccw projected
  arc A162 (-6.0051, 42.0117) -> (-6.6641, 40.4207) centre (-4.4141, 40.4207) ccw projected
  arc A163 (-6.0051, 42.0117) -> (-6.5572, 41.1061) centre (-4.4141, 40.4207) ccw projected
  arc A164 (-6.0051, 42.0117) -> (-6.5572, 41.1061) centre (-4.4141, 40.4207) ccw projected
  line L196 (-4.4141, 40.4207) -> (-6.6641, 40.4207) projected
  line L197 (-6.0051, 42.0117) -> (-4.773, 43.2439) projected
  line L198 (-4.773, 43.2439) -> (-4.5962, 43.0671) projected
  line L199 (-4.4141, 38.1707) -> (-4.4141, 40.4207) projected
  arc A165 (-3.7288, 38.2776) -> (-2.8231, 38.8297) centre (-4.4141, 40.4207) ccw projected
  arc A166 (-3.7288, 38.2776) -> (-2.8231, 38.8297) centre (-4.4141, 40.4207) ccw projected
  arc A167 (-4.4141, 38.1707) -> (-2.8231, 38.8297) centre (-4.4141, 40.4207) ccw projected
  arc A168 (0.9109, 42.9174) -> (-2.8231, 45.1937) centre (-1.2321, 43.6027) ccw projected
  circle A169 centre (-8.4853, 46.9562) radius 5.5 projected
  line L200 (-3.8891, 59.3305) -> (-12.3744, 50.8453) projected
  line L201 (-3.8891, 59.3305) -> (-12.3744, 50.8453) projected
  circle A170 centre (-8.4853, 46.9562) radius 2.5 projected
  line L202 (-10.9853, 46.9562) -> (-13.9853, 46.9562) projected
  circle A171 centre (-8.4853, 46.9562) radius 5.5 projected
  circle A172 centre (-17.1141, 27.7207) radius 6.75 projected
  circle A173 centre (-17.1141, 27.7207) radius 2.5 projected
  line L203 (-13.9853, 14.9482) -> (-13.9853, 21.7397) projected
  line L204 (-13.9853, 14.9482) -> (-13.9853, 21.7397) projected
  circle A174 centre (-17.1141, 27.7207) radius 5.5 projected
  circle A175 centre (-17.1141, 27.7207) radius 2.5 projected
  circle A176 centre (-17.1141, 27.7207) radius 2.5 projected
  line L205 (-17.1141, 27.7207) -> (-17.1141, 15.0207) projected
  line L206 (-17.1141, 27.7207) -> (-17.1141, 15.0207) projected
  circle A177 centre (-17.1141, 15.0207) radius 2.5 projected
  circle A178 centre (-17.1141, 15.0207) radius 2.5 projected
  line L207 (-20.243, 14.9482) -> (-20.243, 21.7397) projected
  line L208 (-20.243, 14.9482) -> (-20.243, 21.7397) projected
  circle A179 centre (-17.1141, 27.7207) radius 2.5 projected
  line L209 (-10.143, 31.5099) -> (-10.8033, 30.8496) projected
  line L210 (-17.1141, 27.7207) -> (-4.4141, 27.7207) projected
  line L211 (-17.1141, 27.7207) -> (-4.4141, 27.7207) projected
  line L212 (2.1213, 30.8496) -> (-11.1331, 30.8496) projected
  line L213 (2.1213, 30.8496) -> (-11.1331, 30.8496) projected
  line L214 (2.1213, 24.5919) -> (-11.1331, 24.5919) projected
  line L215 (5.8389, 53.8558) -> (6.0157, 53.679) projected
  line L216 (0, 55.4415) -> (5.3033, 50.1382) projected
  line L217 (3.3588, 52.0827) -> (8.6914, 57.4153) projected
  circle A180 centre (0, 55.4415) radius 2.5 projected
  circle A181 centre (0, 55.4415) radius 2.5 projected
  circle A182 centre (0, 55.4415) radius 2.5 projected
  circle A183 centre (0, 55.4415) radius 5.5 projected
  circle A184 centre (0, 55.4415) radius 5.5 projected
  line L218 (3.8891, 59.3305) -> (7.2478, 55.9718) projected
  line L219 (0, 55.4415) -> (-3.8891, 59.3305) projected
  circle A185 centre (10.6066, 44.8349) radius 2.5 projected
  circle A186 centre (10.6066, 44.8349) radius 2.5 projected
  line L220 (10.6066, 44.8349) -> (14.4957, 40.9458) projected
  line L221 (14.4957, 40.9458) -> (6.0104, 32.4605) projected
  line L222 (7.2478, 48.1936) -> (5.2873, 46.2331) projected
  line L223 (14.4957, 40.9458) -> (6.0104, 32.4605) projected
  line L224 (6.7175, 48.7239) -> (10.6066, 44.8349) projected
  circle A187 centre (10.6066, 44.8349) radius 5.5 projected
  circle A188 centre (10.6066, 44.8349) radius 2.5 projected
  line L225 (-48.7239, 40.9458) -> (-40.2387, 32.4605) projected
  circle A189 centre (-36.3496, 36.3496) radius 2.5 projected
  circle A190 centre (-36.3496, 36.3496) radius 5.5 projected
  arc A191 (-40.2387, 32.4605) -> (-31.4781, 38.9027) centre (-36.3496, 36.3496) ccw projected
  arc A192 (-40.2387, 32.4605) -> (-31.4781, 38.9027) centre (-36.3496, 36.3496) ccw projected
  line L226 (7.2478, 48.1936) -> (12.5805, 53.5263) projected
  line L227 (12.5805, 53.5263) -> (16.4696, 57.4153) projected
  line L228 (16.4696, 57.4153) -> (12.5805, 61.3044) projected
  line L229 (8.8441, 57.5681) -> (8.6914, 57.4153) projected
  line L230 (12.025, 56.8599) -> (10.0805, 58.8044) projected
  line L231 (12.5805, 61.3044) -> (8.8441, 57.5681) projected
  line L232 (10.0805, 58.8044) -> (13.9696, 54.9153) projected
  line L233 (11.1369, 52.0827) -> (14.4957, 48.7239) projected
  line L234 (16.4696, 57.4153) -> (12.5805, 61.3044) projected
  circle A193 centre (10.6066, 44.8349) radius 5.5 projected
  line L235 (16.4696, 57.4153) -> (23.7174, 50.1675) projected
  line L236 (16.4696, 57.4153) -> (23.7174, 50.1675) projected
  line L237 (14.4957, 40.9458) -> (23.7174, 50.1675) projected
  line L238 (14.4957, 40.9458) -> (23.7174, 50.1675) projected
  line L239 (6.1925, 51.0273) -> (14.525, 59.3599) projected
  arc A194 (6.0104, 22.981) -> (-2.7502, 16.5388) centre (2.1213, 19.0919) ccw projected
  circle A195 centre (2.1213, 19.0919) radius 5.5 projected
  circle A196 centre (2.1213, 36.3496) radius 2.5 projected
  circle A197 centre (2.1213, 36.3496) radius 2.5 projected
  line L240 (-2.8231, 38.8297) -> (-2.7502, 38.9027) projected
  arc A198 (-1.5767, 40.4207) -> (-1.7678, 40.2387) centre (2.1213, 36.3496) ccw projected
  arc A199 (-1.5767, 40.4207) -> (-1.7678, 40.2387) centre (2.1213, 36.3496) ccw projected
  line L241 (-1.7678, 40.2387) -> (-1.2374, 39.7083) projected
  line L242 (-1.591, 40.0619) -> (-1.2321, 40.4207) projected
  circle A200 centre (2.1213, 36.3496) radius 2.5 projected
  line L243 (0.3536, 38.1173) -> (6.0104, 32.4605) projected
  arc A201 (-2.7502, 38.9027) -> (6.0104, 32.4605) centre (2.1213, 36.3496) ccw projected
  arc A202 (-2.7502, 38.9027) -> (6.0104, 32.4605) centre (2.1213, 36.3496) ccw projected
  arc A203 (-2.7502, 38.9027) -> (6.0104, 32.4605) centre (2.1213, 36.3496) ccw projected
  circle A204 centre (2.1213, 36.3496) radius 5.5 projected
  line L244 (-17.1141, 27.7207) -> (-17.1141, 40.4207) projected
  line L245 (-24.0853, 23.9316) -> (-23.425, 24.5919) projected
  line L246 (-20.243, 40.4933) -> (-20.243, 33.7018) projected
  line L247 (-20.243, 46.9562) -> (-20.243, 40.4933) projected
  circle A205 centre (-25.743, 46.9562) radius 5.5 projected
  circle A206 centre (-25.743, 46.9562) radius 2.5 projected
  circle A207 centre (-34.2283, 0) radius 2.5 projected
  circle A208 centre (-25.743, 8.4853) radius 2.5 projected
  circle A209 centre (-34.2283, 0) radius 5.5 projected
  line L248 (-30.3392, -3.8891) -> (-39.5609, -13.1108) projected
  line L249 (-23.243, 8.4853) -> (-20.243, 8.4853) projected
  line L250 (-20.243, 8.4853) -> (-20.243, 14.9482) projected
  circle A210 centre (-25.743, 8.4853) radius 5.5 projected
  line L251 (-30.3392, -3.8891) -> (-21.8539, 4.5962) projected
  line L252 (-20.243, 8.4853) -> (-20.243, 14.9482) projected
  line L253 (-10.9853, 8.4853) -> (-13.9853, 8.4853) projected
  line L254 (-13.9853, 8.4853) -> (-13.9853, 14.9482) projected
  line L255 (-13.9853, 8.4853) -> (-13.9853, 14.9482) projected
  line L256 (-3.8891, -3.8891) -> (-12.3744, 4.5962) projected
  circle A211 centre (-8.4853, 8.4853) radius 2.5 projected
  circle A212 centre (-8.4853, 8.4853) radius 5.5 projected
  line L257 (-17.1141, 27.7207) -> (-29.8141, 27.7207) projected
  line L258 (-36.3496, 30.8496) -> (-23.0952, 30.8496) projected
  line L259 (-17.1141, 27.7207) -> (-29.8141, 27.7207) projected
  line L260 (-36.3496, 24.5919) -> (-23.0952, 24.5919) projected
  circle A213 centre (-36.3496, 19.0919) radius 2.5 projected
  arc A214 (-31.4781, 16.5388) -> (-40.2387, 22.981) centre (-36.3496, 19.0919) ccw projected
  arc A215 (-31.4781, 16.5388) -> (-40.2387, 22.981) centre (-36.3496, 19.0919) ccw projected
  circle A216 centre (-36.3496, 19.0919) radius 5.5 projected
  line L261 (-48.7239, 14.4957) -> (-40.2387, 22.981) projected
  line L262 (-46.8087, -5.863) -> (-39.5609, -13.1108) projected
  line L263 (-50.6978, -1.9739) -> (-46.8087, -5.863) projected
  circle A217 centre (-44.8349, 10.6066) radius 5.5 projected
  line L264 (-50.6978, -1.9739) -> (-57.9457, 5.274) projected
  line L265 (-48.7239, 14.4957) -> (-57.9457, 5.274) projected
  circle A218 centre (-44.8349, 10.6066) radius 2.5 projected
  circle A219 centre (0, 0) radius 2.5 projected
  circle A220 centre (0, 0) radius 5.5 projected
  line L266 (-3.8891, -3.8891) -> (5.3326, -13.1108) projected
  circle A221 centre (2.1213, 19.0919) radius 2.5 projected
  line L267 (14.4957, 14.4957) -> (6.0104, 22.981) projected
  circle A222 centre (10.6066, 10.6066) radius 2.5 projected
  circle A223 centre (10.6066, 10.6066) radius 5.5 projected
  line L268 (14.4957, 14.4957) -> (23.7174, 5.274) projected
  line L269 (16.4696, -1.9739) -> (23.7174, 5.274) projected
  line L270 (16.4696, -1.9739) -> (12.5805, -5.863) projected
  line L271 (12.5805, -5.863) -> (5.3326, -13.1108) projected
  circle A224 centre (-17.1141, 40.4207) radius 2.5 projected
  line L272 (-13.9853, 46.9562) -> (-13.9853, 40.4933) projected
  line L273 (-13.9853, 40.4933) -> (-13.9853, 33.7018) projected
  circle A225 centre (-17.1141, 40.4207) radius 2.5 projected
  line L274 (-20.243, 46.9562) -> (-20.243, 40.4933) projected
  line L275 (-23.243, 46.9562) -> (-20.243, 46.9562) projected
  line L276 (-20.243, 40.4933) -> (-20.243, 33.7018) projected
  line L277 (-24.0853, 31.5099) -> (-23.425, 30.8496) projected
  circle A226 centre (-8.4853, 8.4853) radius 2.5
  circle A227 centre (2.1213, 19.0919) radius 2.5
  circle A228 centre (10.6066, 10.6066) radius 2.5
  circle A229 centre (2.1213, 36.3496) radius 2.5
  circle A230 centre (-8.4853, 46.9562) radius 2.5
  circle A231 centre (10.6066, 44.8349) radius 2.5
  circle A232 centre (0, 55.4415) radius 2.5
  circle A233 centre (-25.743, 46.9562) radius 2.5
  circle A234 centre (-34.2283, 55.4415) radius 2.5
  circle A235 centre (-36.3496, 36.3496) radius 2.5
  circle A236 centre (-44.8349, 44.8349) radius 2.5
  circle A237 centre (-36.3496, 19.0919) radius 2.5
  circle A238 centre (-44.8349, 10.6066) radius 2.5
  circle A239 centre (-34.2283, 0) radius 2.5
  circle A240 centre (-25.743, 8.4853) radius 2.5
  circle A241 centre (0, 0) radius 1.5
  circle A242 centre (10.6066, 10.6066) radius 1.5
  circle A243 centre (2.1213, 19.0919) radius 1.5
  circle A244 centre (-8.4853, 8.4853) radius 1.5
  circle A245 centre (2.1213, 36.3496) radius 1.5
  circle A246 centre (10.6066, 44.8349) radius 1.5
  circle A247 centre (-8.4853, 46.9562) radius 1.5
  circle A248 centre (0, 55.4415) radius 1.5
  circle A249 centre (-34.2283, 0) radius 1.5
  circle A250 centre (-25.743, 8.4853) radius 1.5
  circle A251 centre (-44.9885, 10.6066) radius 1.5
  circle A252 centre (-36.3496, 19.0919) radius 1.5
  circle A253 centre (-36.3496, 36.3496) radius 1.5
  circle A254 centre (-25.743, 46.9562) radius 1.5
  circle A255 centre (-34.2283, 55.4415) radius 1.5
  circle A256 centre (-44.8349, 44.8349) radius 1.5
  circle A257 centre (2.1213, 19.0919) radius 3
  circle A258 centre (10.6066, 10.6066) radius 3
  circle A259 centre (0, 0) radius 3
  circle A260 centre (-8.4853, 8.4853) radius 3
  point P0 (-17.1458, 27.8631)
  point P1 (0.3588, 45.1937)
  point P2 (3.0989, 44.7518)
  point P3 (-5.1265, 43.5974)
  point P4 (-17.1458, 27.8631)
  point P5 (-13.175, 16.6117)
  point P6 (-21.0533, 16.6117)
  point P7 (-21.8539, 4.5962)
  point P8 (-12.3744, 4.5962)
  point P9 (-21.8539, 50.8453)
  point P10 (-21.0533, 38.8297)
  point P11 (8.8441, 4.5909)
  point P12 (8.8441, 4.5909)
  point P13 (0.3588, 13.4297)
  point P14 (-34.5871, 13.4297)
  point P15 (-43.0724, 4.5909)
  point P16 (-43.0724, 4.5909)
  point P17 (6.1925, 4.4141)
  point P18 (8.8441, 4.5909)
  point P19 (-6.0051, 13.4297)
  point P20 (0.3588, 13.4297)
  point P21 (-2.8231, 10.2478)
  point P22 (-43.0724, 50.8506)
  point P23 (-34.5871, 42.0117)
  point P24 (-1.2321, 43.6027)
  point P25 (-6.0051, 42.0117)
  point P26 (0.3588, 45.1937)
  point P27 (0.3588, 42.0117)
  point P28 (-2.8231, 45.1937)
  point P29 (-6.6641, 40.4207)
  point P30 (-6.6641, 40.4207)
  point P31 (-4.4141, 40.4207)
  point P32 (-4.4141, 38.1707)
  dimension "d15" = 5
  dimension "d18" = 3
  dimension "d19" = 3
  dimension "d20" = 3
  dimension "d21" = 3
  dimension "d22" = 3
  dimension "d23" = 3
  dimension "d24" = 3
  dimension "d25" = 3
  dimension "d26" = 3
  dimension "d27" = 3
  dimension "d28" = 3
  dimension "d29" = 3
  dimension "d30" = 3
  dimension "d31" = 3
  dimension "d32" = 3
  dimension "d33" = 3
  dimension "d34" = 6
  dimension "d35" = 6
  dimension "d36" = 6
  dimension "d37" = 6
  constraints: 36 centre point, 34 coincident, 10 concentric, 5 horizontal alignment, 125 other
  measures "d15" diameter of A0
  measures "d18" diameter of A241
  measures "d19" diameter of A242
  measures "d20" diameter of A243
  measures "d21" diameter of A244
  measures "d22" diameter of A245
  measures "d23" diameter of A246
  measures "d24" diameter of A247
  measures "d25" diameter of A248
  measures "d26" diameter of A249
  measures "d27" diameter of A250
  measures "d28" diameter of A251
  measures "d29" diameter of A252
  measures "d30" diameter of A253
  measures "d31" diameter of A254
  measures "d32" diameter of A255
  measures "d33" diameter of A256
  measures "d34" diameter of A257
  measures "d35" diameter of A258
  measures "d36" diameter of A259